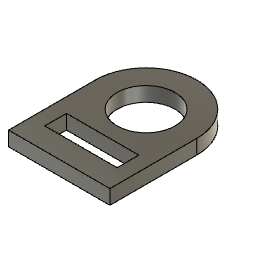
Exercise_1 (Autodesk Fusion 360 design; units mm, degrees)
Autodesk Fusion 360 part; units mm, degrees
sketch "Sketch1" plane through (0, 0, 0) normal (0, 0, 1) x (1, 0, 0)
  line L0 (0, 0) -> (70, 0)
  line L1 (70, 0) -> (70, 60)
  line L2 (55, 60) -> (15, 60)
  line L3 (0, 60) -> (0, 0)
  circle A0 centre (35, 60) radius 20
  arc A1 (70, 60) -> (0, 60) centre (35, 60) ccw
  dimension "d1" = 70
  dimension "d2" = 60
  dimension "d4" = 40
  dimension "d5" = 35
  constraint horizontal L0
  constraint vertical L1
  constraint horizontal L2
  constraint vertical L3
  constraint coincident L0.start L3.end
  constraint concentric A0 A1
  constraint coincident A0 L2.end
  constraint coincident L2 A0.centre
  constraint coincident A0 L2.start
  measures "d1" distance of L0.start L0.end
  measures "d2" distance of L0.start L3.start
  measures "d4" diameter of A0
  measures "d5" radius of A1
sketch "Sketch3" plane through (0, 0, 0) normal (0, 0, 1) x (1, 0, 0)
  line L0 (0, 0) -> (70, 0)
  line L1 (70, 0) -> (70, 60)
  line L2 (0, 60) -> (0, 0)
  arc A0 (70, 60) -> (0, 60) centre (35, 60) ccw
  dimension "d14" = 70
  dimension "d15" = 60
  constraint horizontal L0
  constraint vertical L1
  constraint vertical L2
  constraint coincident L0.start L2.end
  constraint tangent L1 A0
  constraint tangent L2 A0
  measures "d14" distance of L0.start L0.end
  measures "d15" distance of L0.start L2.start
extrude "Extrude3" add sketch "Sketch3" along normal blind 10
hole "Hole1" at (35, 60, 10) direction (0, 0, -1) diameter 40 end through all
sketch "Sketch4" plane through (0, 0, 10) normal (0, 0, 1) x (-1, 0, 0)
  circle A0 centre (-35, -60) radius 20
  arc A1 (-70, -60) -> (0, -60) centre (-35, -60) ccw
  line L0 (0, -60) -> (0, 0)
  line L1 (0, 0) -> (-70, 0)
  line L2 (-70, 0) -> (-70, -60)
  line L3 (-10, -15) -> (-60, -15)
  line L4 (-60, -15) -> (-60, -30)
  line L5 (-60, -30) -> (-10, -30)
  line L6 (-10, -30) -> (-10, -15)
  dimension "d21" = 50
  dimension "d22" = 15
  dimension "d23" = 10
  dimension "d24" = 15
  constraint horizontal L3
  constraint vertical L4
  constraint horizontal L5
  constraint vertical L6
  measures "d21" distance of L3.start L3.end
  measures "d22" distance of L3.start L5.end
  measures "d23" distance of L0 L6
  measures "d24" distance of L1 L3
extrude "Extrude4" cut sketch "Sketch4" against normal through all contours L3 L4 L5 L6
